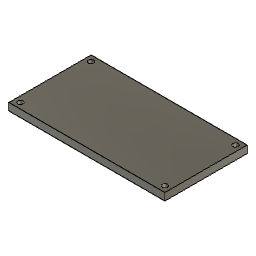
DC Power Converter Board v1 (Autodesk Fusion 360 design; units mm, degrees)
Autodesk Fusion 360 part; units mm, degrees
sketch "Sketch1" plane through (0, 0, 0) normal (0, 0, 1) x (1, 0, 0)
  line L0 (-65, 30) -> (9, 30)
  line L1 (9, 30) -> (9, -9)
  line L2 (9, -9) -> (-65, -9)
  line L3 (-65, -9) -> (-65, 30)
  circle A0 centre (-62.25, 27.25) radius 1.25
  circle A1 centre (6.25, 27.25) radius 1.25
  circle A2 centre (-62.25, -6.25) radius 1.25
  circle A3 centre (6.25, -6.25) radius 1.25
  dimension "d1" = 74
  dimension "d2" = 2.5
  dimension "d3" = 2.5
  dimension "d4" = 2.5
  dimension "d5" = 2.5
  dimension "d6" = 2.75
  dimension "d7" = 39
  dimension "d8" = 2.75
  dimension "d9" = 2.75
  dimension "d10" = 2.75
  dimension "d11" = 2.75
  dimension "d12" = 2.75
  dimension "d13" = 2.75
  dimension "d14" = 2.75
  constraint horizontal L0
  constraint vertical L1
  constraint horizontal L2
  constraint vertical L3
  measures "d1" distance of L0.start L0.end
  measures "d2" diameter of A0
  measures "d3" diameter of A1
  measures "d4" diameter of A2
  measures "d5" diameter of A3
  measures "d6" distance of L0 A0.centre
  measures "d7" distance of L0.end L1.end
  measures "d8" distance of L3 A0.centre
  measures "d9" distance of L0 A1.centre
  measures "d10" distance of L1 A1.centre
  measures "d11" distance of L2 A2.centre
  measures "d12" distance of L3 A2.centre
  measures "d13" distance of L2 A3.centre
  measures "d14" distance of L1 A3.centre
extrude "Extrude1" add sketch "Sketch1" along normal blind 3.5
